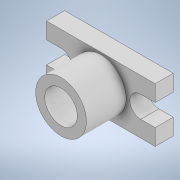
# Autodesk Inventor part: 2-3
Saved by Autodesk Inventor 2020 (Build 240168000, 168)
## iProperties
Created: 2023-11-14
Part Number: 2-3
Material: 常规
Document SubType Name: Modeling
Designer: Z
Density: 1 g/cm^3
Appearance: 默认
Author: Z
Autodesk Inventor part; units mm, degrees
ref_plane "YZ Plane" through (0, 0, 0) normal (1, 0, 0) x (0, 1, 0)
ref_plane "XZ Plane" through (0, 0, 0) normal (0, 1, 0) x (-1, 0, 0)
ref_plane "XY Plane" through (0, 0, 0) normal (0, 0, 1) x (1, 0, 0)
sketch "草图1" plane through (0, 0, 0) normal (0, 0, 1) x (1, 0, 0)
  line L0 (-15, 7.5) -> (15, 7.5)
  line L1 (15, -7.5) -> (-15, -7.5)
  line L2 (-15, 7.5) -> (15, -7.5) construction
  line L3 (15, 7.5) -> (-15, -7.5) construction
  arc A0 (11, 3) -> (11, -3) centre (11, 0) ccw
  arc A1 (-11, -3) -> (-11, 3) centre (-11, 0) ccw
  line L4 (-11, 3) -> (-15, 3)
  line L5 (-11, -3) -> (-15, -3)
  line L6 (11, 3) -> (15, 3)
  line L7 (11, -3) -> (15, -3)
  line L8 (-15, -7.5) -> (-15, -3)
  line L9 (-15, 3) -> (-15, 7.5)
  line L10 (15, 7.5) -> (15, 3)
  line L11 (15, -3) -> (15, -7.5)
  point P0 (0, 0)
  dimension "d0" = 30
  dimension "d1" = 15
  dimension "d4" = 6
  dimension "d5" = 6
  dimension "d6" = 22
  dimension "d7" = 63.435
  dimension "d8" = 63.435
  dimension "d9" = 4.5
  dimension "d10" = 4
  dimension "d11" = 4
  constraints: 24 end point, 6 parallel, 4 perpendicular, 4 point on circle, 4 point on line, 2 centre point, 2 midpoint, 2 tangent, 1 horizontal
  measures "d0" distance of L1.start L1.end
  measures "d1" distance of L0.end L1.start
  measures "d4" diameter of A0
  measures "d5" diameter of A1
  measures "d6" distance of A0.centre A1.centre
  measures "d7" angle of L10 L2
  measures "d8" angle of L10 L3
  measures "d9" distance between parallel lines of L6 L0
  measures "d10" distance from line of L6.start L10
  measures "d11" distance from line of A0.centre L10
extrude "拉伸1" add sketch "草图1" along normal blind 5
sketch "草图2" plane through (0, 0, 5) normal (0, 0, 1) x (1, 0, 0)
  circle A0 centre (0, 0) radius 4.5
  circle A1 centre (0, 0) radius 7
  dimension "d14" = 9
  dimension "d15" = 14
  constraints: 2 centre point, 2 coincident
  measures "d14" diameter of A0
  measures "d15" diameter of A1
extrude "拉伸2" add sketch "草图2" along normal blind 11
